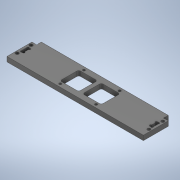
# Autodesk Inventor part: Cockpit_top_frame_
Saved by Autodesk Inventor 2020.4 (Build 244396000, 396)
## iProperties
Created: 2022-01-28
Part Number: Cockpit_top_frame_
Material: アセタール樹脂、黒
Document SubType Name: Modeling
Designer: Masato Kubotera
Density: 1.425 g/cm^3
Appearance: 滑らか - 黒
Author: Masato Kubotera
Autodesk Inventor part; units mm, degrees
ref_plane "YZ Plane" through (0, 0, 0) normal (1, 0, 0) x (0, 1, 0)
ref_plane "XZ Plane" through (0, 0, 0) normal (0, 1, 0) x (-1, 0, 0)
derived "Cockpit_side_frame_.ipt"
sketch "スケッチ2" plane through (0, 0, 0) normal (0, 1, 0) x (-1, 0, 0)
  line L0 (-28.5, -22.5) -> (86.5, -22.5) construction
  line L1 (86.5, -22.5) -> (86.5, -138.5)
  line L2 (86.5, -96) -> (-28.5, -96) construction
  line L3 (-28.5, -96) -> (-28.5, -22.5) construction
  line L4 (-28.5, -22.5) -> (86.5, -96) construction
  line L5 (86.5, -22.5) -> (-28.5, -96) construction
  line L6 (36.5, -101) -> (36.5, -133.5)
  line L7 (41.5, -138.5) -> (86.5, -138.5)
  arc A0 (62.6349, -70.4) -> (61.15, -71.8849) centre (61.8925, -71.1425) ccw
  arc A1 (71.15, -72.5349) -> (69.6651, -71.05) centre (70.4075, -71.7925) ccw
  line L8 (63.3349, -71.05) -> (69.6651, -71.05)
  line L9 (62.6349, -70.4) -> (70.3651, -70.4)
  line L10 (61.9, -71.1) -> (71.1, -71.1) construction
  arc A2 (63.3349, -71.05) -> (61.85, -72.5349) centre (62.5925, -71.7925) ccw
  line L11 (61.2, -70.45) -> (71.8, -70.45) construction
  line L12 (71.15, -72.5349) -> (71.15, -83.4651)
  line L13 (71.8, -78) -> (61.2, -78) construction
  line L14 (71.85, -71.8849) -> (71.85, -84.1151)
  line L15 (71.1, -71.1) -> (71.1, -84.9) construction
  line L16 (61.85, -72.5349) -> (61.85, -83.4651)
  line L17 (71.8, -70.45) -> (71.8, -85.55) construction
  line L18 (61.15, -71.8849) -> (61.15, -84.1151)
  line L19 (66.5, -70.45) -> (66.5, -85.55) construction
  line L20 (61.9, -84.9) -> (61.9, -71.1) construction
  line L21 (71.1, -71.1) -> (61.9, -84.9) construction
  line L22 (71.8, -70.45) -> (61.2, -85.55) construction
  line L23 (61.2, -70.45) -> (71.8, -85.55) construction
  line L24 (61.2, -85.55) -> (61.2, -70.45) construction
  line L25 (61.9, -71.1) -> (71.1, -84.9) construction
  arc A3 (71.85, -71.8849) -> (70.3651, -70.4) centre (71.1075, -71.1425) ccw
  line L26 (71.1, -84.9) -> (61.9, -84.9) construction
  line L27 (71.8, -85.55) -> (61.2, -85.55) construction
  arc A4 (61.85, -83.4651) -> (63.3349, -84.95) centre (62.5925, -84.2075) ccw
  arc A5 (61.15, -84.1151) -> (62.6349, -85.6) centre (61.8925, -84.8575) ccw
  line L28 (63.3349, -84.95) -> (69.6651, -84.95)
  line L29 (62.6349, -85.6) -> (70.3651, -85.6)
  arc A6 (69.6651, -84.95) -> (71.15, -83.4651) centre (70.4075, -84.2075) ccw
  arc A7 (70.3651, -85.6) -> (71.85, -84.1151) centre (71.1075, -84.8575) ccw
  line L30 (-23.5, -22.5) -> (-28.5, -27.5)
  line L31 (-28.5, -59.25) -> (86.5, -59.25) construction
  line L32 (29, -22.5) -> (29, -96) construction
  line L33 (-23.5, -96) -> (-28.5, -91)
  line L34 (-28.5, -27.5) -> (-28.5, -91)
  line L35 (-21, -25) -> (-26, -25) construction
  line L36 (-26, -25) -> (-26, -93.5) construction
  line L37 (-26, -93.5) -> (-21, -93.5) construction
  line L38 (-21, -93.5) -> (-21, -25) construction
  line L39 (-21, -25) -> (-26, -93.5) construction
  line L40 (-26, -25) -> (-21, -93.5) construction
  line L41 (-26.05, -46.7) -> (-20.95, -46.7)
  line L42 (-20.95, -46.7) -> (-20.95, -71.8)
  line L43 (-20.95, -71.8) -> (-26.05, -71.8)
  line L44 (-26.05, -71.8) -> (-26.05, -46.7)
  line L45 (-26.05, -46.7) -> (-20.95, -71.8) construction
  line L46 (-20.95, -46.7) -> (-26.05, -71.8) construction
  line L47 (-26, -46.75) -> (-21, -46.75) construction
  line L48 (-26, -71.75) -> (-21, -71.75) construction
  line L49 (-23.5, -25) -> (-23.5, -93.5) construction
  circle A8 centre (-23.5, -35) radius 3
  circle A9 centre (-23.5, -35) radius 1.6
  arc A10 (-24.5651, -46.7) -> (-26.05, -48.1849) centre (-25.3075, -47.4425) ccw
  arc A11 (-20.95, -48.1849) -> (-22.4349, -46.7) centre (-21.6925, -47.4425) ccw
  arc A12 (-22.4349, -71.8) -> (-20.95, -70.3151) centre (-21.6925, -71.0575) ccw
  arc A13 (-26.05, -70.3151) -> (-24.5651, -71.8) centre (-25.3075, -71.0575) ccw
  circle A14 centre (-23.5, -83.5) radius 1.6
  circle A15 centre (-23.5, -83.5) radius 3
  line L50 (31.5, -96) -> (36.5, -101)
  line L51 (-23.5, -96) -> (31.5, -96)
  line L52 (79, -67.5) -> (-21, -67.5) construction
  line L53 (-21, -67.5) -> (-21, -62.5) construction
  line L54 (-21, -62.5) -> (79, -62.5) construction
  line L55 (79, -62.5) -> (79, -67.5) construction
  line L56 (79, -67.5) -> (-21, -62.5) construction
  line L57 (-21, -67.5) -> (79, -62.5) construction
  line L58 (-21, -65) -> (79, -65) construction
  line L59 (29, -62.5) -> (29, -67.5) construction
  line L60 (4, -62.5) -> (4, -67.5) construction
  line L61 (54.05, -62.45) -> (3.95, -62.45)
  line L62 (3.95, -62.45) -> (3.95, -67.55)
  line L63 (3.95, -67.55) -> (54.05, -67.55)
  line L64 (54.05, -67.55) -> (54.05, -62.45)
  line L65 (54.05, -62.45) -> (3.95, -67.55) construction
  line L66 (3.95, -62.45) -> (54.05, -67.55) construction
  arc A16 (5.4349, -62.45) -> (3.95, -63.9349) centre (4.6925, -63.1925) ccw
  circle A17 centre (-3.5, -65) radius 3
  circle A18 centre (-3.5, -65) radius 1.6
  line L67 (54, -62.5) -> (54, -67.5) construction
  arc A19 (54.05, -63.9349) -> (52.5651, -62.45) centre (53.3075, -63.1925) ccw
  circle A20 centre (61.5, -65) radius 3
  circle A21 centre (61.5, -65) radius 1.6
  arc A22 (3.95, -66.0651) -> (5.4349, -67.55) centre (4.6925, -66.8075) ccw
  arc A23 (52.5651, -67.55) -> (54.05, -66.0651) centre (53.3075, -66.8075) ccw
  line L68 (-21, -88.5) -> (79, -88.5) construction
  line L69 (79, -88.5) -> (79, -93.5) construction
  line L70 (79, -93.5) -> (-21, -93.5) construction
  line L71 (-21, -93.5) -> (-21, -88.5) construction
  line L72 (-21, -88.5) -> (79, -93.5) construction
  line L73 (79, -88.5) -> (-21, -93.5) construction
  line L74 (-21, -91) -> (79, -91) construction
  line L75 (29, -88.5) -> (29, -93.5) construction
  line L76 (54.05, -91.05) -> (3.95, -91.05)
  line L77 (3.95, -91.05) -> (3.95, -88.45)
  line L78 (3.95, -88.45) -> (54.05, -88.45)
  line L79 (54.05, -88.45) -> (54.05, -91.05)
  line L80 (54.05, -91.05) -> (3.95, -88.45) construction
  line L81 (3.95, -91.05) -> (54.05, -88.45) construction
  line L82 (4, -88.5) -> (4, -91) construction
  line L83 (54, -88.5) -> (54, -91) construction
  line L84 (4, -89.75) -> (54, -89.75) construction
  arc A24 (6.05, -88.45) -> (3.95, -88.45) centre (5, -88.45) ccw
  arc A25 (54.05, -88.45) -> (51.95, -88.45) centre (53, -88.45) ccw
  arc A26 (51.95, -91.05) -> (54.05, -91.05) centre (53, -91.05) ccw
  arc A27 (3.95, -91.05) -> (6.05, -91.05) centre (5, -91.05) ccw
  circle A28 centre (-3.5, -91) radius 3
  circle A29 centre (-3.5, -91) radius 1.6
  circle A30 centre (61.5, -91) radius 3 construction
  circle A31 centre (61.5, -91) radius 1.6 construction
  line L85 (-23.5, -22.5) -> (64.25, -22.5)
  line L86 (64.25, -22.5) -> (64.25, -17.5)
  line L87 (64.25, -17.5) -> (72.25, -17.5)
  line L88 (72.25, -17.5) -> (72.25, -22.5)
  line L89 (72.25, -22.5) -> (79, -22.5)
  line L90 (79, -22.5) -> (79, -17.5)
  line L91 (86.5, -22.5) -> (86.5, -20)
  line L92 (79, -17.5) -> (84, -17.5)
  line L93 (84, -17.5) -> (86.5, -20)
  line L94 (68.25, -17.5) -> (68.25, -22.5) construction
  arc A32 (62.7651, -22.5) -> (64.25, -21.0151) centre (63.5075, -21.7575) ccw
  arc A33 (72.25, -21.0151) -> (73.7349, -22.5) centre (72.9925, -21.7575) ccw
  arc A34 (77.5151, -22.5) -> (79, -21.0151) centre (78.2575, -21.7575) ccw
  line L95 (-16, -88.5) -> (-16, -68.5) construction
  line L96 (-16, -68.5) -> (64, -68.5) construction
  line L97 (64, -68.5) -> (64, -88.5) construction
  line L98 (45.5, -86) -> (-16.5, -86)
  line L99 (-18.5, -84) -> (-18.5, -72)
  line L100 (-16.5, -70) -> (45.5, -70)
  line L101 (47.5, -72) -> (47.5, -84)
  line L102 (47.5, -86) -> (-18.5, -70) construction
  line L103 (-18.5, -86) -> (47.5, -70) construction
  arc A35 (-16.5, -70) -> (-18.5, -72) centre (-16.5, -72) ccw
  arc A36 (-18.5, -84) -> (-16.5, -86) centre (-16.5, -84) ccw
  arc A37 (45.5, -86) -> (47.5, -84) centre (45.5, -84) ccw
  arc A38 (47.5, -72) -> (45.5, -70) centre (45.5, -72) ccw
  line L104 (36.5, -133.5) -> (41.5, -138.5)
  line L105 (44, -131) -> (39, -131) construction
  line L106 (39, -131) -> (39, -96) construction
  line L107 (39, -96) -> (44, -96) construction
  line L108 (44, -96) -> (44, -131) construction
  line L109 (44, -131) -> (39, -96) construction
  line L110 (39, -131) -> (44, -96) construction
  line L111 (41.5, -96) -> (41.5, -131) construction
  line L112 (39, -113.5) -> (44, -113.5) construction
  line L113 (41.5, -107.5) -> (44, -107.5) construction
  line L114 (41.45, -107.45) -> (44.05, -107.45)
  line L115 (44.05, -107.45) -> (44.05, -119.55)
  line L116 (44.05, -119.55) -> (41.45, -119.55)
  line L117 (41.45, -119.55) -> (41.45, -107.45)
  line L118 (41.45, -107.45) -> (44.05, -119.55) construction
  line L119 (44.05, -107.45) -> (41.45, -119.55) construction
  arc A39 (44.05, -109.55) -> (44.05, -107.45) centre (44.05, -108.5) ccw
  arc A40 (42.9349, -107.45) -> (41.45, -108.9349) centre (42.1925, -108.1925) ccw
  arc A41 (44.05, -119.55) -> (44.05, -117.45) centre (44.05, -118.5) ccw
  line L120 (41.5, -119.5) -> (44, -119.5) construction
  arc A42 (41.45, -118.0651) -> (42.9349, -119.55) centre (42.1925, -118.8075) ccw
  line L121 (42.75, -107.5) -> (42.75, -119.5) construction
  circle A43 centre (41.5, -125.5) radius 3 construction
  circle A44 centre (41.5, -125.5) radius 1.6 construction
  circle A45 centre (41.5, -101.5) radius 3
  circle A46 centre (41.5, -101.5) radius 1.6
  circle A47 centre (-13.5, -55) radius 2
  line L122 (39, -131) -> (77.8645, -131) construction
  line L123 (77.8645, -131) -> (77.8645, -136) construction
  line L124 (77.8645, -136) -> (39, -136) construction
  line L125 (39, -136) -> (39, -131) construction
  line L126 (39, -131) -> (77.8645, -136) construction
  line L127 (77.8645, -131) -> (39, -136) construction
  line L128 (39, -133.5) -> (77.8645, -133.5) construction
  line L129 (58.4322, -131) -> (58.4322, -136) construction
  line L130 (58.4322, -133.5) -> (58.4322, -131) construction
  line L131 (50.8822, -130.95) -> (65.9822, -130.95)
  line L132 (65.9822, -130.95) -> (65.9822, -133.55)
  line L133 (65.9822, -133.55) -> (50.8822, -133.55)
  line L134 (50.8822, -133.55) -> (50.8822, -130.95)
  line L135 (50.8822, -130.95) -> (65.9822, -133.55) construction
  line L136 (65.9822, -130.95) -> (50.8822, -133.55) construction
  line L137 (50.9322, -131) -> (50.9322, -133.5) construction
  arc A48 (52.9822, -130.95) -> (50.8822, -130.95) centre (51.9322, -130.95) ccw
  arc A49 (50.8822, -132.0651) -> (52.3672, -133.55) centre (51.6247, -132.8075) ccw
  arc A50 (65.9822, -130.95) -> (63.8822, -130.95) centre (64.9322, -130.95) ccw
  arc A51 (64.4973, -133.55) -> (65.9822, -132.0651) centre (65.2398, -132.8075) ccw
  line L138 (65.9322, -131) -> (65.9322, -133.5) construction
  line L139 (50.9322, -132.25) -> (65.9322, -132.25) construction
  circle A52 centre (72.4322, -133.5) radius 1.6 construction
  circle A53 centre (72.4322, -133.5) radius 3 construction
  circle A54 centre (44.4322, -133.5) radius 3
  circle A55 centre (44.4322, -133.5) radius 1.6
  line L140 (48.5, -96) -> (77, -96)
  line L141 (79, -98) -> (79, -126.5)
  line L142 (77, -128.5) -> (48.5, -128.5)
  line L143 (46.5, -126.5) -> (46.5, -98)
  line L144 (46.5, -96) -> (79, -128.5) construction
  line L145 (79, -96) -> (46.5, -128.5) construction
  arc A56 (48.5, -96) -> (46.5, -98) centre (48.5, -98) ccw
  arc A57 (46.5, -126.5) -> (48.5, -128.5) centre (48.5, -126.5) ccw
  arc A58 (77, -128.5) -> (79, -126.5) centre (77, -126.5) ccw
  arc A59 (79, -98) -> (77, -96) centre (77, -98) ccw
  line L146 (79, -91.1738) -> (84, -91.1738) construction
  line L147 (84, -91.1738) -> (84, -136) construction
  line L148 (84, -136) -> (79, -136) construction
  line L149 (79, -136) -> (79, -91.1738) construction
  line L150 (79, -91.1738) -> (84, -136) construction
  line L151 (84, -91.1738) -> (79, -136) construction
  line L152 (81.5, -91.1738) -> (81.5, -136) construction
  circle A60 centre (81.5, -93.6738) radius 1.475
  circle A61 centre (81.5, -98.6738) radius 1.475
  circle A62 centre (81.5, -103.6738) radius 1.475
  circle A63 centre (81.5, -133.5) radius 1.6
  arc A64 (84, -91.1738) -> (79, -91.1738) centre (81.5, -133.5) ccw construction
  arc A65 (84.0111, -91.0742) -> (78.9889, -91.0742) centre (81.5, -133.5) ccw construction
  line L153 (86.5, -133.5) -> (81.5, -138.5)
  arc A66 (79, -131) -> (84, -136) centre (81.5, -133.5) ccw construction
  line L154 (79, -65) -> (84, -65) construction
  line L155 (84, -65) -> (84, -91) construction
  line L156 (84, -91) -> (79, -91) construction
  line L157 (79, -91) -> (79, -65) construction
  line L158 (79, -65) -> (84, -91) construction
  line L159 (84, -65) -> (79, -91) construction
  line L160 (79, -78) -> (84, -78) construction
  line L161 (81.5, -65) -> (81.5, -91) construction
  line L162 (79, -73) -> (84, -73) construction
  line L163 (78.95, -72.95) -> (86.5, -72.95)
  line L164 (84.05, -72.95) -> (84.05, -83.05) construction
  line L165 (84.05, -83.05) -> (78.95, -83.05)
  line L166 (78.95, -83.05) -> (78.95, -72.95)
  line L167 (78.95, -72.95) -> (84.05, -83.05) construction
  line L168 (84.05, -72.95) -> (78.95, -83.05) construction
  arc A67 (80.4349, -72.95) -> (78.95, -74.4349) centre (79.6925, -73.6925) ccw
  arc A68 (78.95, -81.5651) -> (80.4349, -83.05) centre (79.6925, -82.3075) ccw
  line L169 (79, -83) -> (84, -83) construction
  circle A69 centre (81.5, -68) radius 1.6
  circle A70 centre (81.5, -68) radius 3
  circle A71 centre (81.5, -88) radius 1.6
  circle A72 centre (81.5, -88) radius 3
  line L170 (84.05, -83.05) -> (86.5, -83.05)
  circle A73 centre (81.5, -133.5) radius 3
  line L171 (75.625, -22.5) -> (75.625, -27.147) construction
  line L172 (60.875, -22.5) -> (60.875, -27.147) construction
  line L173 (64.25, -22.5) -> (72.25, -22.5)
  point P0 (0, 0)
  point P1 (29, -59.25)
  point P2 (-25.7227, -96)
  point P3 (61.85, -71.05)
  point P4 (61.15, -70.4)
  point P5 (66.5, -78)
  point P6 (-23.5, -59.25)
  point P7 (29, -65)
  point P8 (29, -91)
  point P9 (29, -89.75)
  point P10 (29, -89.75)
  point P11 (52.5, -22)
  point P12 (14.5, -78)
  point P13 (-18.5, -61)
  point P14 (47.5, -61)
  point P15 (41.5, -113.5)
  point P16 (42.75, -113.5)
  point P17 (58.4322, -133.5)
  point P18 (58.4322, -132.25)
  point P19 (62.75, -112.25)
  point P20 (81.5, -113.5869)
  point P21 (81.5, -78)
  dimension "d1" = 22.5
  dimension "d2" = 5
  measures "d1" vertical distance of L0.end point (0, 0)
  measures "d2" vertical distance of L0.end L92.end
ref_plane "作業平面1" through (0, 0, -22.5) normal (0, 0, 1) x (1, 0, 0)
sketch "スケッチ3" plane through (0, 0, -22.5) normal (0, 0, 1) x (1, 0, 0)
  line L0 (-84, -140) -> (-52.5, -140)
  line L1 (-52.5, -140) -> (-52.5, 5)
  line L2 (-52.5, 5) -> (-84, 5)
  line L3 (-84, 5) -> (-84, -140)
  line L4 (-84, -140) -> (-52.5, 5) construction
  line L5 (-52.5, -140) -> (-84, 5) construction
  line L6 (-72.25, 2.5) -> (-64.25, 2.5) construction
  line L7 (-64.25, 2.5) -> (-64.25, 0) construction
  line L8 (-64.25, 0) -> (-72.25, 0) construction
  line L9 (-72.25, 0) -> (-72.25, 2.5) construction
  line L10 (-72.25, 2.5) -> (-64.25, 0) construction
  line L11 (-64.25, 2.5) -> (-72.25, 0) construction
  line L12 (-79.05, 5) -> (-79.05, 0)
  line L13 (-79.05, 0) -> (-84, 0)
  arc A0 (-80.5349, 0) -> (-79.05, 1.4849) centre (-79.7925, 0.7425) ccw
  line L14 (-72.3, 2.55) -> (-64.2, 2.55)
  line L15 (-64.2, 2.55) -> (-64.2, -0.05)
  line L16 (-64.2, -0.05) -> (-72.3, -0.05)
  line L17 (-72.3, -0.05) -> (-72.3, 2.55)
  line L18 (-72.3, 2.55) -> (-64.2, -0.05) construction
  line L19 (-64.2, 2.55) -> (-72.3, -0.05) construction
  line L20 (-72.25, 1.25) -> (-64.25, 1.25) construction
  line L21 (-68.25, 2.5) -> (-68.25, 0) construction
  arc A1 (-70.8151, 2.55) -> (-72.3, 1.0651) centre (-71.5575, 1.8075) ccw
  arc A2 (-72.3, -0.05) -> (-70.2, -0.05) centre (-71.25, -0.05) ccw
  arc A3 (-64.2, 1.0651) -> (-65.6849, 2.55) centre (-64.9425, 1.8075) ccw
  arc A4 (-66.3, -0.05) -> (-64.2, -0.05) centre (-65.25, -0.05) ccw
  line L22 (-58.9, -64.85) -> (-77.6, -64.85) construction
  line L23 (-77.6, -64.85) -> (-77.6, -46.15) construction
  line L24 (-77.6, -46.15) -> (-58.9, -46.15) construction
  line L25 (-58.9, -46.15) -> (-58.9, -64.85) construction
  line L26 (-58.9, -64.85) -> (-77.6, -46.15) construction
  line L27 (-77.6, -64.85) -> (-58.9, -46.15) construction
  line L28 (-68.25, -55.5) -> (-68.25, -79.5) construction
  line L29 (-60.3142, -45.5642) -> (-76.1858, -45.5642)
  line L30 (-78.1858, -47.5642) -> (-78.1858, -63.4358)
  line L31 (-76.1858, -65.4358) -> (-60.3142, -65.4358)
  line L32 (-58.3142, -63.4358) -> (-58.3142, -47.5642)
  line L33 (-58.3142, -45.5642) -> (-78.1858, -65.4358) construction
  line L34 (-78.1858, -45.5642) -> (-58.3142, -65.4358) construction
  arc A5 (-58.3142, -47.5642) -> (-60.3142, -45.5642) centre (-60.3142, -47.5642) ccw
  arc A6 (-76.1858, -45.5642) -> (-78.1858, -47.5642) centre (-76.1858, -47.5642) ccw
  arc A7 (-78.1858, -63.4358) -> (-76.1858, -65.4358) centre (-76.1858, -63.4358) ccw
  arc A8 (-60.3142, -65.4358) -> (-58.3142, -63.4358) centre (-60.3142, -63.4358) ccw
  line L35 (-55.75, -48.5) -> (-80.75, -48.5) construction
  line L36 (-80.75, -48.5) -> (-80.75, -86.5) construction
  line L37 (-80.75, -86.5) -> (-55.75, -86.5) construction
  line L38 (-55.75, -86.5) -> (-55.75, -48.5) construction
  line L39 (-55.75, -48.5) -> (-80.75, -86.5) construction
  line L40 (-80.75, -48.5) -> (-55.75, -86.5) construction
  circle A9 centre (-55.75, -48.5) radius 1.25
  circle A10 centre (-80.75, -48.5) radius 1.25
  line L41 (-84, -67.5) -> (-52.5, -67.5)
  circle A11 centre (-75.625, 2.5) radius 1.6
  circle A12 centre (-60.875, 2.5) radius 1.6
  point P0 (0, 0)
  point P1 (-68.25, -67.5)
  point P2 (-52.5, 0)
  point P3 (-68.25, 1.25)
  point P4 (-79, 0)
  point P5 (-79, 0)
  point P6 (-79, 0)
  point P7 (-68.25, -67.5)
  point P8 (-68.25, -67.5)
  point P9 (-68.25, -67.5)
  point P10 (-66.3, -0.05)
  point P11 (-65.6849, 2.55)
  point P12 (-64.2, 1.0651)
  point P13 (-75.625, 0)
  point P14 (-75.625, 0)
  point P15 (-60.875, 0)
  point P16 (-60.875, 0)
  point P17 (-60.875, 0)
  dimension "d4" = 5
  dimension "d5" = 145
  dimension "d6" = 2.5
  dimension "d7" = 0.05
  dimension "d8" = 1.05
  dimension "d9" = 0.05
  dimension "d10" = 0.05
  dimension "d11" = 1.05
  dimension "d12" = 1.05
  dimension "d13" = 18.7
  dimension "d14" = 18.7
  dimension "d15" = 24
  dimension "d16" = 2
  dimension "d17" = 25
  dimension "d18" = 38
  dimension "d19" = 2.5
  dimension "d20" = 2.5
  dimension "d24" = 3.2
  dimension "d25" = 14.75
  dimension "d26" = 14.75
  constraints: 84 end point, 23 midpoint, 22 point on circle, 19 point on line, 13 centre point, 12 parallel, 8 tangent, 7 perpendicular, 6 horizontal, 6 symmetric about line, 3 coincident, 3 equal radius, 2 vertical, 3 other
  measures "d4" distance of L2.end L13.end
  measures "d5" distance of L0.end L1.end
  measures "d6" distance of L8.end L6.start
  measures "d7" distance of L12.end point (-79, 0)
  measures "d8" radius of A0
  measures "d9" horizontal distance of L14.start L6.start
  measures "d10" horizontal distance of L14.start L6.start
  measures "d11" radius of A1
  measures "d12" radius of A2
  measures "d13" distance of L24.end L23.end
  measures "d14" distance of L22.end L23.end
  measures "d15" distance of L28.start L28.end
  measures "d16" radius of A5
  measures "d17" distance of L38.start L36.end
  measures "d18" distance of L36.end L36.start
  measures "d19" diameter of A9
  measures "d20" diameter of A10
  measures "d24" diameter of A11
  measures "d25" distance of point (-75.625, 0) point (-60.875, 0)
  measures "d26" distance of A12.centre A11.centre
extrude "押し出し1" add sketch "スケッチ3" along normal blind 5 contours L3 L13 A0 L12 L2 L1 L41
mirror "ミラー1" about plane through (-84, -67.5, -22.5) normal (0, -1, 0)
equation "\"d9\" = d7"
equation "\"d10\" = d9"
equation "\"d12\" = d11"
equation "\"d13\" = d14"
equation "\"d20\" = d19"
equation "\"d26\" = d25"
equation "\"d3\" = -d1"
